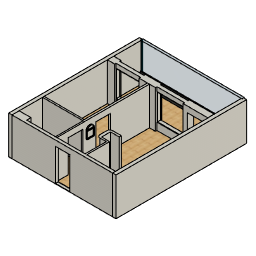
OmaSpace (Autodesk Fusion 360 design; units mm, degrees)
Autodesk Fusion 360 part; units mm, degrees
note: some values were not read from the file. Chosen so that the rebuilt part matches the saved one: which bodies a step acts on.
sketch "Sketch1" plane through (0, 0, 0) normal (0, 0, 1) x (1, 0, 0)
  line L0 (-3708.5119, 4762.4356) -> (3649.0423, 4762.4356)
  line L1 (3649.0423, 4762.4356) -> (3649.0423, -4198.8685)
  line L2 (3649.0423, -4198.8685) -> (-3708.5119, -4198.8685)
  line L3 (-3708.5119, -4198.8685) -> (-3708.5119, 4762.4356)
  line L4 (-3483.4242, 2778.8502) -> (3400, 2778.8502)
  line L5 (3400, 2778.8502) -> (3400, 4650)
  line L6 (3400, 4650) -> (-3483.4242, 4650)
  line L7 (-3483.4242, 4650) -> (-3483.4242, 2778.8502)
  line L8 (-3483.4242, 2345.186) -> (-734.9519, 2345.186)
  line L9 (-734.9519, 2345.186) -> (-734.9519, -1993.9055)
  line L10 (-734.9519, -1993.9055) -> (-3483.4242, -1993.9055)
  line L11 (-3483.4242, -1993.9055) -> (-3483.4242, 2345.186)
  line L12 (-599.7778, 2345.186) -> (3414.8957, 2345.186)
  line L13 (3414.8957, 2345.186) -> (3414.8957, -1683.0048)
  line L14 (3414.8957, -1683.0048) -> (-599.7778, -1683.0048)
  line L15 (-599.7778, -1683.0048) -> (-599.7778, 2345.186)
  line L16 (3414.8957, -1683.0048) -> (1500, -1683.0048)
  line L17 (1500, -1683.0048) -> (1500, -4000)
  line L18 (1500, -4000) -> (3414.8957, -4000)
  line L19 (3414.8957, -4000) -> (3414.8957, -1683.0048)
  line L20 (1444.7568, -2414.12) -> (1500, -2414.12)
  line L21 (1500, -2414.12) -> (1500, -4000)
  line L22 (1500, -4000) -> (1444.7568, -4000)
  line L23 (1444.7568, -4000) -> (1444.7568, -2414.12)
  line L24 (-599.7778, -1683.0048) -> (700, -1683.0048)
  line L25 (700, -1683.0048) -> (700, -4000)
  line L26 (700, -4000) -> (-599.7778, -4000)
  line L27 (-599.7778, -4000) -> (-599.7778, -1683.0048)
  line L28 (700, -4000) -> (1334.6921, -4000)
  line L29 (1334.6921, -4000) -> (1334.6921, -2552.7927)
  line L30 (1334.6921, -2552.7927) -> (700, -2552.7927)
  line L31 (700, -2552.7927) -> (700, -4000)
  line L32 (-3483.4242, -2106.3353) -> (-700, -2106.3353)
  line L33 (-700, -2106.3353) -> (-700, -4000)
  line L34 (-700, -4000) -> (-3483.4242, -4000)
  line L35 (-3483.4242, -4000) -> (-3483.4242, -2106.3353)
  line L36 (-3483.4242, -3707.9425) -> (-2668.5277, -3707.9425)
  line L37 (-2668.5277, -3707.9425) -> (-2668.5277, -4000)
  line L38 (-2668.5277, -4000) -> (-3483.4242, -4000) construction
  line L39 (-3483.4242, -4000) -> (-3483.4242, -3707.9425) construction
  line L40 (-2984.5775, 2778.8502) -> (-1317.2599, 2778.8502)
  line L41 (-1317.2599, 2778.8502) -> (-1317.2599, 2345.186)
  line L42 (-1317.2599, 2345.186) -> (-2984.5775, 2345.186)
  line L43 (-2984.5775, 2345.186) -> (-2984.5775, 2778.8502)
  line L44 (-189.543, 2778.8502) -> (1699.764, 2778.8502)
  line L45 (1699.764, 2778.8502) -> (1699.764, 2345.186)
  line L46 (1699.764, 2345.186) -> (-189.543, 2345.186)
  line L47 (-189.543, 2345.186) -> (-189.543, 2778.8502)
  line L48 (1918.2058, 2778.8502) -> (2916.248, 2778.8502)
  line L49 (2916.248, 2778.8502) -> (2916.248, 2345.186)
  line L50 (2916.248, 2345.186) -> (1918.2058, 2345.186)
  line L51 (1918.2058, 2345.186) -> (1918.2058, 2778.8502)
  line L52 (1918.2058, 2687.0366) -> (2916.248, 2687.0366)
  line L53 (2916.248, 2687.0366) -> (2916.248, 2446.706)
  line L54 (2916.248, 2446.706) -> (1918.2058, 2446.706)
  line L55 (1918.2058, 2446.706) -> (1918.2058, 2687.0366)
  line L56 (-189.543, 2689.8655) -> (1699.764, 2689.8655)
  line L57 (1699.764, 2689.8655) -> (1699.764, 2446.706)
  line L58 (1699.764, 2446.706) -> (-189.543, 2446.706)
  line L59 (-189.543, 2446.706) -> (-189.543, 2689.8655)
  line L60 (-2984.5775, 2681.7776) -> (-1317.2599, 2681.7776)
  line L61 (-1317.2599, 2681.7776) -> (-1317.2599, 2438.4627)
  line L62 (-1317.2599, 2438.4627) -> (-2984.5775, 2438.4627)
  line L63 (-2984.5775, 2438.4627) -> (-2984.5775, 2681.7776)
  line L64 (-3527, 4808.2914) -> (3450, 4808.2914)
  line L65 (3450, 4808.2914) -> (3450, 4650)
  line L66 (3450, 4650) -> (-3527, 4650)
  line L67 (-3527, 4650) -> (-3527, 4808.2914)
  line L68 (-734.9519, -398.1035) -> (-599.7778, -398.1035)
  line L69 (-599.7778, -398.1035) -> (-599.7778, -1278.0251)
  line L70 (-599.7778, -1278.0251) -> (-734.9519, -1278.0251)
  line L71 (-734.9519, -1278.0251) -> (-734.9519, -398.1035)
  line L72 (-734.9519, -328.9773) -> (-599.7778, -328.9773)
  line L73 (-599.7778, -328.9773) -> (-599.7778, -1340.5015)
  line L74 (-599.7778, -1340.5015) -> (-734.9519, -1340.5015)
  line L75 (-734.9519, -1340.5015) -> (-734.9519, -328.9773)
  line L76 (-700, -2200) -> (-599.7778, -2200)
  line L77 (-599.7778, -2200) -> (-599.7778, -3216.879)
  line L78 (-599.7778, -3216.879) -> (-700, -3216.879)
  line L79 (-700, -3216.879) -> (-700, -2200)
  line L80 (-700, -3146.0723) -> (-599.7778, -3146.0723)
  line L81 (-599.7778, -3146.0723) -> (-599.7778, -2266.0462)
  line L82 (-599.7778, -2266.0462) -> (-700, -2266.0462)
  line L83 (-700, -2266.0462) -> (-700, -3146.0723)
  line L84 (-500, -4000) -> (473.9143, -4000)
  line L85 (473.9143, -4000) -> (473.9143, -4198.8685)
  line L86 (473.9143, -4198.8685) -> (-500, -4198.8685)
  line L87 (-500, -4198.8685) -> (-500, -4000)
  line L88 (-451.6304, -4000) -> (423.3381, -4000)
  line L89 (423.3381, -4000) -> (423.3381, -4198.8685)
  line L90 (423.3381, -4198.8685) -> (-451.6304, -4198.8685)
  line L91 (-451.6304, -4198.8685) -> (-451.6304, -4000)
  line L92 (899.8143, -1828.3915) -> (1500, -1828.3915)
  line L93 (1500, -1828.3915) -> (1500, -2437.0798)
  line L94 (1500, -2437.0798) -> (899.8143, -2437.0798)
  line L95 (899.8143, -2437.0798) -> (899.8143, -1828.3915)
  line L96 (-3483.4242, 4591.2856) -> (3400, 4591.2856)
  dimension "d1" = 6977
  constraint horizontal L0
  constraint vertical L1
  constraint horizontal L2
  constraint vertical L3
  constraint horizontal L4
  constraint vertical L5
  constraint horizontal L6
  constraint vertical L7
  constraint horizontal L8
  constraint vertical L9
  constraint horizontal L10
  constraint vertical L11
  constraint horizontal L12
  constraint vertical L13
  constraint horizontal L14
  constraint vertical L15
  constraint horizontal L16
  constraint vertical L17
  constraint horizontal L18
  constraint vertical L19
  constraint horizontal L20
  constraint vertical L21
  constraint horizontal L22
  constraint vertical L23
  constraint horizontal L24
  constraint vertical L25
  constraint horizontal L26
  constraint vertical L27
  constraint horizontal L28
  constraint vertical L29
  constraint horizontal L30
  constraint vertical L31
  constraint horizontal L32
  constraint vertical L33
  constraint horizontal L34
  constraint vertical L35
  constraint horizontal L36
  constraint vertical L37
  constraint horizontal L38
  constraint vertical L39
  constraint coincident L34 L37.end
  constraint coincident L35 L36.start
  constraint horizontal L40
  constraint vertical L41
  constraint horizontal L42
  constraint vertical L43
  constraint coincident L8 L41.end
  constraint coincident L4 L40.start
  constraint horizontal L44
  constraint vertical L45
  constraint horizontal L46
  constraint vertical L47
  constraint coincident L12 L45.end
  constraint coincident L4 L44.start
  constraint horizontal L48
  constraint vertical L49
  constraint horizontal L50
  constraint vertical L51
  constraint coincident L12 L49.end
  constraint horizontal L52
  constraint vertical L53
  constraint horizontal L54
  constraint vertical L55
  constraint coincident L49 L53.end
  constraint coincident L51 L52.start
  constraint horizontal L56
  constraint vertical L57
  constraint horizontal L58
  constraint vertical L59
  constraint coincident L45 L57.end
  constraint coincident L47 L56.start
  constraint horizontal L60
  constraint vertical L61
  constraint horizontal L62
  constraint vertical L63
  constraint coincident L41 L61.end
  constraint coincident L43 L60.start
  constraint horizontal L64
  constraint vertical L65
  constraint horizontal L66
  constraint vertical L67
  constraint horizontal L68
  constraint vertical L69
  constraint horizontal L70
  constraint vertical L71
  constraint coincident L15 L69.end
  constraint coincident L9 L68.start
  constraint horizontal L72
  constraint vertical L73
  constraint horizontal L74
  constraint vertical L75
  constraint coincident L15 L73.end
  constraint coincident L9 L72.start
  constraint horizontal L76
  constraint vertical L77
  constraint horizontal L78
  constraint vertical L79
  constraint coincident L27 L77.end
  constraint coincident L33 L76.start
  constraint horizontal L80
  constraint vertical L81
  constraint horizontal L82
  constraint vertical L83
  constraint coincident L77 L81.end
  constraint coincident L79 L80.start
  constraint horizontal L84
  constraint vertical L85
  constraint horizontal L86
  constraint vertical L87
  constraint coincident L2 L85.end
  constraint coincident L26 L84.start
  constraint horizontal L88
  constraint vertical L89
  constraint horizontal L90
  constraint vertical L91
  constraint coincident L86 L89.end
  constraint coincident L26 L88.start
  constraint horizontal L92
  constraint vertical L93
  constraint horizontal L94
  constraint vertical L95
  constraint coincident L21 L93.end
  constraint coincident L7 L96.start
  constraint coincident L5 L96.end
  constraint perpendicular L5 L96
  measures "d1" distance of L65 L67
extrude "Extrude21" add sketch "Sketch1" along normal blind 1 makes body 1
extrude "Extrude19" add sketch "Sketch1" along normal blind 800 separate body contours L5 L6 L7 L66 L96 makes body 2
extrude "Extrude15" add sketch "Sketch1" along normal blind 2600 separate body contours L41 L43 L60 L61 L62 L63 makes body 3
extrude "Extrude14" add sketch "Sketch1" along normal blind 2600 separate body contours L0 L1 L2 L4 L5 L12 L13 L14 L17 L18 L19 L22 L23 L25 L26 L28 L29 L30 L49 L53 L65 L66 L85 L92 L94 L95 | L4 L48 L49 L51 L52 | L4 L8 L9 L12 L15 L41 L47 L59 L61 L72 | L4 L12 L45 L51 L55 L57 | L49 L51 L52 L53 L54 L55 | L12 L49 L50 L51 L54 | L45 L47 L56 L57 L58 L59 makes body 4
extrude "Extrude13" add sketch "Sketch1" along normal blind 2600 separate body contours L0 L64 L65 L67 | L0 L6 L65 L66 L67 makes body 5
extrude "Extrude7" add sketch "Sketch1" along normal blind 2600 separate body contours L0 L2 L3 L4 L7 L8 L9 L10 L11 L15 L26 L27 L32 L33 L34 L35 L43 L63 L66 L67 L74 L76 L78 L87 | L2 L26 L84 L86 L87 L91 | L2 L26 L84 L86 L88 L89 L90 L91 | L2 L26 L84 L85 L86 L89 | L27 L33 L77 L78 L79 L80 | L27 L33 L77 L79 L80 L81 L82 L83 | L27 L33 L76 L77 L79 L82 | L34 L35 L36 L37 | L9 L15 L70 L73 L74 L75 | L9 L15 L68 L69 L70 L71 L73 L75 | L9 L15 L68 L72 L73 L75 makes body 6
sketch "Sketch2" plane through (0, 2345.186, 0) normal (0, -1, 0) x (1, 0, 0)
  line L0 (1699.764, 0) -> (3414.8957, 0)
  line L1 (3414.8957, 0) -> (3414.8957, 2600)
  line L2 (3414.8957, 2600) -> (1699.764, 2600)
  line L3 (1699.764, 2600) -> (1699.764, 0)
  line L4 (2000, 0) -> (3000, 0)
  line L5 (3000, 0) -> (3000, 2200)
  line L6 (3000, 2200) -> (2000, 2200)
  line L7 (2000, 2200) -> (2000, 0)
  dimension "d16" = 1000
  dimension "d17" = 2200
  constraint horizontal L4
  constraint vertical L5
  constraint horizontal L6
  constraint vertical L7
  constraint coincident L0 L4.start
  measures "d16" distance of L4.start L4.end
  measures "d17" distance of L4.end L5.end
extrude "Extrude17" cut sketch "Sketch2" against normal blind 500 contours L0 L4 L5 L6 L7 bodies 4
sketch "Sketch3" plane through (-599.7778, 0, 0) normal (1, 0, 0) x (0, 1, 0)
  line L0 (-4000, 0) -> (-328.9773, 0)
  line L1 (-328.9773, 0) -> (-328.9773, 2600)
  line L2 (-328.9773, 2600) -> (-4000, 2600)
  line L3 (-4000, 2600) -> (-4000, 0)
  line L4 (-328.9773, 0) -> (-1328.9773, 0)
  line L5 (-1328.9773, 0) -> (-1328.9773, 2200)
  line L6 (-1328.9773, 2200) -> (-328.9773, 2200)
  line L7 (-328.9773, 2200) -> (-328.9773, 0)
  line L8 (-3220.0462, 0) -> (-2220.0462, 0)
  line L9 (-2220.0462, 0) -> (-2220.0462, 2200)
  line L10 (-2220.0462, 2200) -> (-3220.0462, 2200)
  line L11 (-3220.0462, 2200) -> (-3220.0462, 0)
  dimension "d20" = 1000
  dimension "d21" = 2200
  dimension "d22" = 1000
  dimension "d23" = 2200
  constraint horizontal L4
  constraint vertical L5
  constraint horizontal L6
  constraint vertical L7
  constraint coincident L0.end L1.start
  constraint horizontal L8
  constraint vertical L9
  constraint horizontal L10
  constraint vertical L11
  constraint coincident L0 L8.start
  measures "d20" distance of L0.end L4.end
  measures "d21" distance of L0.end L6.end
  measures "d22" distance of L8.start L8.end
  measures "d23" distance of L8.start L10.end
extrude "Extrude9" cut sketch "Sketch3" against normal blind 500 contours L0 L8 L9 L10 L11 | L0 L1 L4 L5 L6 L7 bodies 6
sketch "Sketch4" plane through (0, 2438.4627, 0) normal (0, -1, 0) x (1, 0, 0)
  line L0 (-2984.5775, 0) -> (-1317.2599, 0)
  line L1 (-1317.2599, 0) -> (-1317.2599, 2600)
  line L2 (-1317.2599, 2600) -> (-2984.5775, 2600)
  line L3 (-2984.5775, 2600) -> (-2984.5775, 0)
  line L4 (-2984.5775, 494.4633) -> (-1317.2599, 494.4633)
  line L5 (-1317.2599, 494.4633) -> (-1317.2599, 2294.4633)
  line L6 (-1317.2599, 2294.4633) -> (-2984.5775, 2294.4633)
  line L7 (-2984.5775, 2294.4633) -> (-2984.5775, 494.4633)
  line L8 (-1337.2599, 514.4633) -> (-1337.2599, 2274.4633)
  line L9 (-1337.2599, 2274.4633) -> (-2964.5775, 2274.4633)
  line L10 (-2964.5775, 2274.4633) -> (-2964.5775, 514.4633)
  line L11 (-2964.5775, 514.4633) -> (-1337.2599, 514.4633)
  line L12 (-2964.5775, 514.4633) -> (-1337.2599, 514.4633)
  line L13 (-1337.2599, 514.4633) -> (-1337.2599, 2274.4633)
  line L14 (-1337.2599, 2274.4633) -> (-2964.5775, 2274.4633)
  line L15 (-2964.5775, 2274.4633) -> (-2964.5775, 514.4633)
  dimension "d26" = 1800
  dimension "d65" = -20
  dimension "d75" = -20
  constraint horizontal L4
  constraint vertical L5
  constraint horizontal L6
  constraint vertical L7
  constraint coincident L3 L4.start
  measures "d26" distance of L4.start L6.end
extrude "Extrude24" cut sketch "Sketch4" against normal blind 10 contours L1 L3 L4 L5 L6 L7 bodies 3
extrude "Extrude23" cut sketch "Sketch4" against normal blind 300 contours L8 L9 L10 L11 L12 L13 L14 L15 bodies 3
sketch "Sketch5" plane through (0, 2446.706, 0) normal (0, -1, 0) x (1, 0, 0)
  line L0 (-189.543, 0) -> (1699.764, 0)
  line L1 (1699.764, 0) -> (1699.764, 2600)
  line L2 (1699.764, 2600) -> (-189.543, 2600)
  line L3 (-189.543, 2600) -> (-189.543, 0)
  line L4 (-189.543, 2295.8957) -> (-189.543, 495.8957)
  line L5 (-189.543, 495.8957) -> (1699.764, 495.8957)
  line L6 (1699.764, 495.8957) -> (1699.764, 2295.8957)
  line L7 (1699.764, 2295.8957) -> (-189.543, 2295.8957)
  line L8 (-189.543, 2295.8957) -> (-189.543, 495.8957)
  line L9 (-169.543, 515.8957) -> (1679.764, 515.8957)
  line L10 (1679.764, 515.8957) -> (1679.764, 2275.8957)
  line L11 (1679.764, 2275.8957) -> (-169.543, 2275.8957)
  line L12 (-169.543, 2275.8957) -> (-169.543, 515.8957)
  dimension "d31" = 1800
  dimension "d70" = -20
  constraint vertical L4
  constraint coincident L3 L4.end
  constraint horizontal L5
  constraint vertical L6
  constraint horizontal L7
  constraint vertical L8
  measures "d31" distance of L4.end L4.start
extrude "Extrude25" cut sketch "Sketch5" against normal blind 20 contours L1 L3 L4 L5 L6 L7 L8 bodies 4
fillet "Fillet1" radius 200 1 edges at (700, -1683.0048, 1300) on bodies 4
fillet "Fillet2" radius 200 1 edges at (700, -2552.7927, 1300) on bodies 4
sketch "Sketch6" plane through (-599.7778, 0, 0) normal (1, 0, 0) x (0, 1, 0)
  line L0 (-328.9773, 0) -> (2345.186, 0)
  line L1 (2345.186, 0) -> (2345.186, 2600)
  line L2 (2345.186, 2600) -> (-328.9773, 2600)
  line L3 (-328.9773, 2600) -> (-328.9773, 0)
  line L4 (-2000, 2000) -> (-1500, 2000)
  line L5 (-1500, 2000) -> (-1500, 1500)
  line L6 (-1500, 1500) -> (-2000, 1500)
  line L7 (-2000, 1500) -> (-2000, 2000)
  arc A0 (-1500, 2000) -> (-2000, 2000) centre (-1750, 2000) ccw
  line L8 (-1510, 1990) -> (-1510, 1510)
  line L9 (-1510, 1510) -> (-1990, 1510)
  line L10 (-1990, 1510) -> (-1990, 1990)
  line L11 (-1990, 1990) -> (-1510, 1990)
  arc A1 (-1510, 2000) -> (-1990, 2000) centre (-1750, 2000) ccw
  dimension "d53" = 500
  dimension "d54" = 500
  dimension "d55" = 10
  dimension "d56" = -10
  constraint horizontal L4
  constraint vertical L5
  constraint horizontal L6
  constraint vertical L7
  constraint tangent L5 A0
  measures "d53" distance of L4.start L4.end
  measures "d54" distance of L4.start L6.end
extrude "Extrude20" add sketch "Sketch6" along normal blind 80 contours L4 A0 A1 | L4 L5 L6 L7 bodies 6
ref_plane "WorkPlane1" through (-1617.2988, -4198.8685, 1300) normal (0, -1, 0) x (1, 0, 0)
sketch "Sketch7" plane through (-1617.2988, -4198.8685, 1300) normal (0, -1, 0) x (1, 0, 0)
  line L0 (1120.169, -1275.6249) -> (2100, -1275.6249)
  line L1 (2100, -1275.6249) -> (2100, 924.3751)
  line L2 (2100, 924.3751) -> (1120.169, 924.3751)
  line L3 (1120.169, 924.3751) -> (1120.169, -1275.6249)
  dimension "d62" = 2200
  constraint horizontal L0
  constraint vertical L1
  constraint horizontal L2
  constraint vertical L3
  measures "d62" distance of L0.start L2.end
extrude "Extrude22" cut sketch "Sketch7" against normal blind 300 bodies 4 6
extrude "Extrude26" cut 1 faces at (1063.3284, 2446.706, 1102.5623) along direction (0, 1, 0) up to surface (243.1595 mm away) on bodies 4 bodies 4
ref_plane "WorkPlane2" through (3414.8957, -827.407, 1300) normal (-1, 0, 0) x (0, -1, 0)
split "Split1" by plane through (3414.8957, -827.407, 1300) normal (-1, 0, 0) bodies 4 makes body 7 at (2437.4975, -4198.8685, 1608.125) makes body 8 at (-599.7778, 562.4105, 866.6667)
ref_plane "WorkPlane3" through (-3483.4242, 175.6403, 1300) normal (1, 0, 0) x (0, 1, 0)
split "Split2" by plane through (-3483.4242, 175.6403, 1300) normal (1, 0, 0) bodies 6 makes body 9 at (-3317.1419, 2778.8502, 866.6667) makes body 10 at (-2487.9927, -4198.8685, 1608.125)
combine "Combine1" operation add target body 10 tool bodies 7
ref_plane "WorkPlane4" through (-34.2642, -4000.0005, 1300) normal (0, -1, 0) x (1, 0, 0)
split "Split3" by plane through (-34.2642, -4000.0005, 1300) normal (0, -1, 0) bodies 10 makes body 11 at (-2487.9927, -4198.8685, 1608.125)
ref_plane "WorkPlane5" through (-599.7778, -2164.4886, 1300) normal (1, 0, 0) x (0, 1, 0)
split "Split4" by plane through (-599.7778, -2164.4886, 1300) normal (1, 0, 0) bodies 10 makes body 12 at (2437.4975, -4000.0005, 1608.125) makes body 13 at (-546.4444, -1614.3634, 2210.0065)
ref_plane "WorkPlane6" through (-394.6604, 2345.186, 1300) normal (0, -1, 0) x (1, 0, 0)
split "Split5" by plane through (-394.6604, 2345.186, 1300) normal (0, -1, 0) bodies 8 makes body 14 at (-599.7778, 562.4105, 866.6667)
ref_plane "WorkPlane7" through (-734.9519, -1161.4414, 1300) normal (-1, 0, 0) x (0, -1, 0)
split "Split6" by plane through (-734.9519, -1161.4414, 1300) normal (-1, 0, 0) bodies 10 makes body 15 at (-2567.2668, -2106.3353, 866.6667) makes body 16 at (-1651.1094, -4000.0005, 1733.3333)
combine "Combine2" operation add target body 16 tool bodies 11
combine "Combine3" operation add target body 14 tool bodies 10
combine "Combine4" operation add target body 3 tool bodies 8
ref_plane "WorkPlane8" through (3400, 3714.4251, 1300) normal (-1, 0, 0) x (0, -1, 0)
split "Split7" by plane through (3400, 3714.4251, 1300) normal (-1, 0, 0) bodies 3 makes body 17 at (-941.3543, 2778.8502, 866.6667)
combine "Combine5" operation add target body 3 tool bodies 4
combine "Combine6" operation add target body 12 tool bodies 16
combine "Combine7" operation add target body 9 tool bodies 17
sketch "Sketch8" plane through (-3483.4242, 0, 0) normal (1, 0, 0) x (0, 1, 0)
  line L0 (-4198.8685, 0) -> (4650, 0)
  line L1 (4650, 0) -> (4650, 2600)
  line L2 (4650, 2600) -> (-4198.8685, 2600)
  line L3 (-4198.8685, 2600) -> (-4198.8685, 0)
named bodies: "LeftWall", "BelconyGlass", "RightWall", "BelconyButtom", "Floor", "RightWall (1)", "RightWall (2)", "Wall", "LeftWall (2)", "LeftWall (2) (1)", "FrontWall", "Decoration", "Mid-Wall", "LeftMidWall", "LeftWall (2) (5)"
